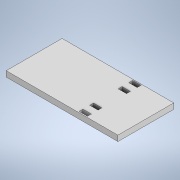
# Autodesk Inventor part: main_base
Saved by Autodesk Inventor 2022 (Build 260153000, 153)
## iProperties
Created: 2022-02-02
Part Number: main_base
Material: Generic
Document SubType Name: Modeling
Designer: Iñigo
Density: 1 g/cm^3
Appearance: Default
Author: Iñigo
Autodesk Inventor part; units mm, degrees
ref_plane "YZ Plane" through (0, 0, 0) normal (1, 0, 0) x (0, 1, 0)
ref_plane "XZ Plane" through (0, 0, 0) normal (0, 1, 0) x (-1, 0, 0)
ref_plane "XY Plane" through (0, 0, 0) normal (0, 0, 1) x (1, 0, 0)
sketch "Sketch1" plane through (0, 0, 0) normal (0, 1, 0) x (-1, 0, 0)
  line L0 (-100, 50) -> (100, 50)
  line L1 (100, 50) -> (100, -50)
  line L2 (100, -50) -> (-100, -50)
  line L3 (-100, -50) -> (-100, 50)
  line L4 (-100, 50) -> (100, -50) construction
  line L5 (100, 50) -> (-100, -50) construction
  point P0 (0, 0)
  dimension "d0" = 200
  dimension "d1" = 100
  constraints: 12 end point, 2 midpoint, 2 parallel, 1 horizontal, 1 perpendicular
  measures "d0" distance of L1.end L2.end
  measures "d1" distance of L0.end L1.end
extrude "Extrusion1" add sketch "Sketch1" along normal blind 10
sketch "Sketch2" plane through (0, 10, 0) normal (0, 1, 0) x (1, 0, 0)
  line L0 (43.4356, -48) -> (28.4356, -48)
  line L1 (28.4356, -48) -> (28.4356, -41)
  line L2 (28.4356, -41) -> (43.4356, -41)
  line L3 (43.4356, -41) -> (43.4356, -48)
  line L4 (-100, -50) -> (100, -50) projected
  line L5 (24.9047, 0) -> (58.9924, 0)
  line L6 (25.9332, -35) -> (42.5456, -35)
  line L7 (43.4356, -22) -> (28.4356, -22)
  line L8 (28.4356, -22) -> (28.4356, -29)
  line L9 (28.4356, -29) -> (43.4356, -29)
  line L10 (43.4356, -29) -> (43.4356, -22)
  line L11 (43.4356, 48) -> (28.4356, 48)
  line L12 (28.4356, 48) -> (28.4356, 41)
  line L13 (28.4356, 41) -> (43.4356, 41)
  line L14 (43.4356, 41) -> (43.4356, 48)
  line L15 (43.4356, 29) -> (43.4356, 22)
  line L16 (43.4356, 22) -> (28.4356, 22)
  line L17 (28.4356, 22) -> (28.4356, 29)
  line L18 (28.4356, 29) -> (43.4356, 29)
  point P0 (0, 0)
  dimension "d5" = 15
  dimension "d6" = 7
  dimension "d11" = 2
  dimension "d12" = 6
  constraints: 36 end point, 12 symmetric about line, 3 horizontal, 2 parallel, 1 perpendicular
  measures "d5" distance of L1.end L2.end
  measures "d6" distance of L0.end L1.end
  measures "d11" distance between parallel lines of L0 L4
  measures "d12" distance between parallel lines of L6 L2
extrude "Extrusion2" cut sketch "Sketch2" against normal blind 25
body "Solid1"
